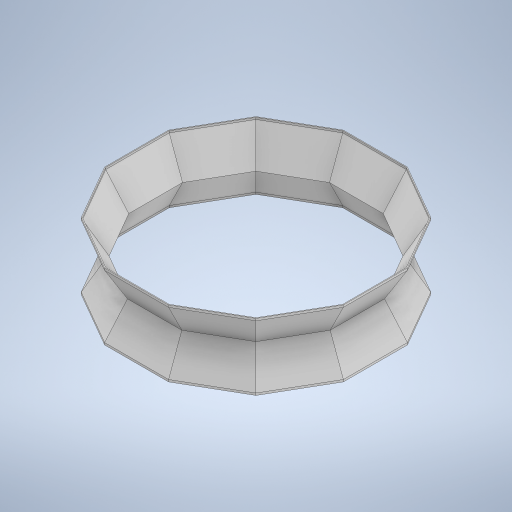
# Autodesk Inventor part: OV-PAM_n_12_standard_1F
Saved by Autodesk Inventor 2024 (Build 280153000, 153)
## iProperties
Created: 2023-08-31
Part Number: OV-PAM_n_12_standard_1F
Material: 일반
Document SubType Name: Modeling
Designer: jsw
Density: 1 g/cm^3
Appearance: 기본값
Author: jsw
Autodesk Inventor part; units mm, degrees
ref_plane "YZ Plane" through (0, 0, 0) normal (1, 0, 0) x (0, 1, 0)
sketch "스케치1" plane through (0, 0, 0) normal (0, 1, 0) x (-1, 0, 0)
  line L0 (-18.2607, 68.1499) -> (18.2607, 68.1499)
  line L1 (18.2607, 68.1499) -> (49.8892, 49.8892)
  line L2 (49.8892, 49.8892) -> (68.1499, 18.2607)
  line L3 (68.1499, 18.2607) -> (68.1499, -18.2607)
  line L4 (68.1499, -18.2607) -> (49.8892, -49.8892)
  line L5 (49.8892, -49.8892) -> (18.2607, -68.1499)
  line L6 (18.2607, -68.1499) -> (-18.2607, -68.1499)
  line L7 (-18.2607, -68.1499) -> (-49.8892, -49.8892)
  line L8 (-49.8892, -49.8892) -> (-68.1499, -18.2607)
  line L9 (-68.1499, -18.2607) -> (-68.1499, 18.2607)
  line L10 (-68.1499, 18.2607) -> (-49.8892, 49.8892)
  line L11 (-49.8892, 49.8892) -> (-18.2607, 68.1499)
  line L12 (18.4215, -68.7499) -> (-18.4215, -68.7499)
  line L13 (-18.4215, -68.7499) -> (-50.3284, -50.3284)
  line L14 (-50.3284, -50.3284) -> (-68.7499, -18.4215)
  line L15 (-68.7499, -18.4215) -> (-68.7499, 18.4215)
  line L16 (-68.7499, 18.4215) -> (-50.3284, 50.3284)
  line L17 (-50.3284, 50.3284) -> (-18.4215, 68.7499)
  line L18 (-18.4215, 68.7499) -> (18.4215, 68.7499)
  line L19 (18.4215, 68.7499) -> (50.3284, 50.3284)
  line L20 (50.3284, 50.3284) -> (68.7499, 18.4215)
  line L21 (68.7499, 18.4215) -> (68.7499, -18.4215)
  line L22 (68.7499, -18.4215) -> (50.3284, -50.3284)
  line L23 (50.3284, -50.3284) -> (18.4215, -68.7499)
  point P0 (0, 0)
  point P1 (0, 0)
  point P2 (0, 0)
  dimension "d1" = 141.108
  dimension "d2" = 0.6
  constraints: 48 end point, 2 coincident, 2 horizontal, 50 other
  measures "d1" distance of L8.end L2.end
  measures "d2" distance between parallel lines of L3 L21
extrude "돌출1" add sketch "스케치1" along normal blind 18 contours L0 L1 L2 L3 L4 L5 L6 L7 L8 L9 L10 L11 | L12 L13 L14 L15 L16 L17 L18 L19 L20 L21 L22 L23
ref_plane "작업 평면1" through (50.3284, 0, 50.3284) normal (-0.75, -0.5, -0.4330127) x (0.5, 0, -0.8660254)
sketch "스케치2" plane through (68.7499, 0, 18.4215) normal (0.8660254, 0, 0.5) x (0.5, 0, -0.8660254)
  line L0 (-36.843, 0) -> (0, 0) projected
  line L1 (0, 0) -> (0, 18) projected
  line L2 (-36.843, 18) -> (0, 18) projected
  line L3 (-36.843, 0) -> (-36.843, 18) projected
  line L4 (-36.843, 0) -> (-68.7499, 0) projected
  line L5 (-36.843, 0) -> (-68.0199, 18)
  line L6 (-36.843, 18) -> (-68.7499, 18) projected
  line L7 (0, 0) -> (-1, 18)
  line L8 (-36.843, 18) -> (-68.0199, 18)
  point P0 (-18.4215, 0)
  point P1 (-34.675, 12)
  dimension "d6" = 150
  dimension "d7" = 1
  constraints: 6 end point, 2 point on line, 1 collinear
  measures "d6" angle of L5 L0
  measures "d7" distance of L1.end L7.end
extrude "돌출2" cut sketch "스케치2" against normal up to surface surface through (50.3284, 0, 50.3284) normal (-0.75, -0.5, -0.4330127)
pattern_circular "원형 패턴1" count 12 over 360 about axis through (0, -10, 0) along (0, 1, 0) of "돌출2"
sketch "스케치3" plane through (0, 0, 0) normal (0, -1, 0) x (1, 0, 0)
  line L0 (-50.3284, -50.3284) -> (-68.7499, -18.4215) projected
  line L1 (-18.4215, -68.7499) -> (-50.3284, -50.3284) projected
  line L2 (18.4215, -68.7499) -> (-18.4215, -68.7499) projected
  line L3 (50.3284, -50.3284) -> (18.4215, -68.7499) projected
  line L4 (68.7499, -18.4215) -> (50.3284, -50.3284) projected
  line L5 (68.7499, 18.4215) -> (68.7499, -18.4215) projected
  line L6 (50.3284, 50.3284) -> (68.7499, 18.4215) projected
  line L7 (18.4215, 68.7499) -> (50.3284, 50.3284) projected
  line L8 (-18.4215, 68.7499) -> (18.4215, 68.7499) projected
  line L9 (-50.3284, 50.3284) -> (-18.4215, 68.7499) projected
  line L10 (-68.7499, 18.4215) -> (-50.3284, 50.3284) projected
  line L11 (-68.7499, -18.4215) -> (-68.7499, 18.4215) projected
  point P0 (0, 0)
extrude "돌출3" add sketch "스케치3" along normal blind 1.2
ref_plane "작업 평면2" through (0, 18, 0) normal (0, 1, 0) x (1, 0, 0)
mirror "미러1" about plane through (0, 18, 0) normal (0, 1, 0) of "돌출2", "원형 패턴1", "돌출3", "돌출1"
shell "쉘1" thickness 0.5 removed faces 2 at (10.6357, 37.2, -6.1405) at (10.6357, -1.2, -6.1405)
